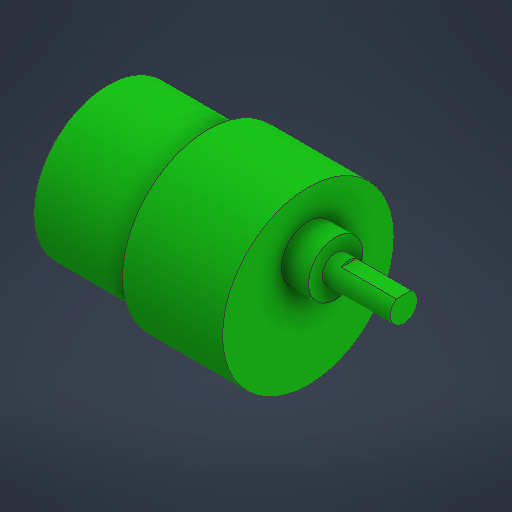
# Autodesk Inventor part: Drive Motor approximate
Saved by Autodesk Inventor 2026.2 (Build 302298010, 298A)
## iProperties
Created: 2026-06-06
Part Number: Drive Motor approximate
Material: Generic
Document SubType Name: Modeling
Designer: Inigo Greenall
Density: 1 g/cm^3
Appearance: Default
Author: Inigo Greenall
Autodesk Inventor part; units mm, degrees
ref_plane "YZ Plane" through (0, 0, 0) normal (1, 0, 0) x (0, 1, 0)
ref_plane "XZ Plane" through (0, 0, 0) normal (0, 1, 0) x (-1, 0, 0)
ref_plane "XY Plane" through (0, 0, 0) normal (0, 0, 1) x (1, 0, 0)
sketch "Sketch1" plane through (0, 0, 0) normal (1, 0, 0) x (0, 1, 0)
  circle A0 centre (0, 0) radius 16.35
  dimension "d0" = 32.7
  constraints: 1 centre point, 1 coincident
  measures "d0" diameter of A0
extrude "Extrusion1" add sketch "Sketch1" along normal blind 22
sketch "Sketch2" plane through (22, 0, 0) normal (1, 0, 0) x (0, 0, -1)
  circle A0 centre (0, 0) radius 18.85
  dimension "d3" = 37.7
  constraints: 1 centre point, 1 coincident
  measures "d3" diameter of A0
extrude "Extrusion2" add sketch "Sketch2" along normal blind 22
sketch "Sketch3" plane through (44, 0, 0) normal (1, 0, 0) x (0, 0, -1)
  circle A0 centre (0, 6.4) radius 5.95
  circle A1 centre (0, 0) radius 18.85 projected
  line L0 (0, 18.85) -> (0, 12.35) construction
  dimension "d8" = 11.9
  dimension "d7" = 6.5
  constraints: 3 vertical alignment, 2 end point, 1 point on line, 1 vertical, 3 other
  measures "d7" distance of L0.start L0.end
extrude "Extrusion3" add sketch "Sketch3" along normal blind 6 contours A0
sketch "Sketch4" plane through (50, 6.4, 0) normal (1, 0, 0) x (0, 0, -1)
  circle A0 centre (0, 0) radius 5.95 projected
  circle A1 centre (0, 0) radius 3
  point P0 (0, -6.4)
  dimension "d14" = 6
  constraints: 1 centre point, 1 coincident
  measures "d14" diameter of A1
extrude "Extrusion4" add sketch "Sketch4" along normal blind 15 contours A1
sketch "Sketch5" plane through (65, 6.4, 0) normal (1, 0, 0) x (0, 0, -1)
  circle A0 centre (0, 0) radius 3 projected
  line L0 (-1.6583, 2.5) -> (1.6583, 2.5)
  point P0 (0, 2.5)
  dimension "d17" = 2.5
  constraints: 2 end point, 2 point on circle, 1 horizontal, 1 midpoint
  measures "d17" distance of A0.centre point (0, 2.5)
extrude "Extrusion5" cut sketch "Sketch5" against normal blind 12.1 contours L0 A0 picked at (-0.1169, 2.6598)
body "Solid1"
